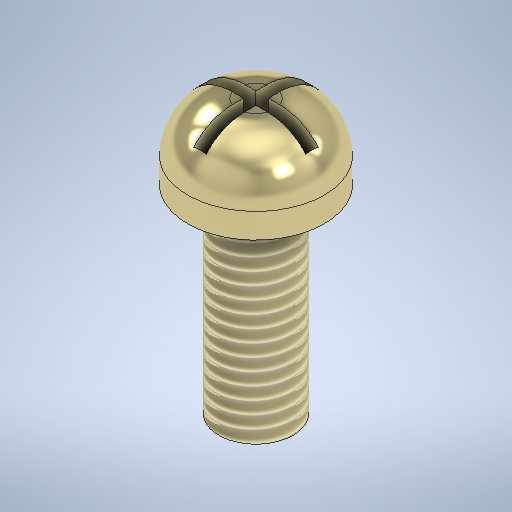
# Autodesk Inventor part: M3 Schraube
Saved by Autodesk Inventor 2025.1 (Build 291241000, 241)
## iProperties
Created: 2024-12-19
Part Number: M3 Schraube
Material: Generisch
Document SubType Name: Modeling
Designer: Julian
Density: 1 g/cm^3
Appearance: Vorgabe
Author: Julian
Autodesk Inventor part; units mm, degrees
ref_plane "YZ Plane" through (0, 0, 0) normal (1, 0, 0) x (0, 1, 0)
ref_plane "XZ Plane" through (0, 0, 0) normal (0, 1, 0) x (-1, 0, 0)
ref_plane "XY Plane" through (0, 0, 0) normal (0, 0, 1) x (1, 0, 0)
sketch "Skizze1" plane through (0, 0, 0) normal (0, 0, 1) x (1, 0, 0)
  circle A0 centre (0, 0) radius 2.75
  dimension "d0" = 5.5
  constraints: 1 centre point, 1 coincident
  measures "d0" diameter of A0
extrude "Extrusion1" add sketch "Skizze1" along normal blind 3
fillet "Rundung1" radius 2 1 edges at (-2.75, 0, 3)
sketch "Skizze2" plane through (0, 0, 3) normal (0, 0, 1) x (1, 0, 0)
  line L0 (0.25, -2.25) -> (-0.25, -2.25)
  line L1 (-0.25, 2.25) -> (0.25, 2.25)
  line L2 (0.25, -2.25) -> (-0.25, 2.25) construction
  line L3 (-0.25, -2.25) -> (0.25, 2.25) construction
  line L4 (-2.25, 0.25) -> (-2.25, -0.25)
  line L5 (2.25, -0.25) -> (2.25, 0.25)
  line L6 (2.25, 0.25) -> (-2.25, -0.25) construction
  line L7 (-2.25, 0.25) -> (2.25, -0.25) construction
  line L8 (-0.25, 0.25) -> (-2.25, 0.25)
  line L9 (-0.25, 0.25) -> (-0.25, 2.25)
  line L10 (-0.25, -2.25) -> (-0.25, -0.25)
  line L11 (-0.25, -0.0278) -> (-0.25, 0.0278)
  line L12 (2.25, 0.25) -> (0.25, 0.25)
  line L13 (0.0278, 0.25) -> (-0.0278, 0.25)
  line L14 (0.25, -0.25) -> (2.25, -0.25)
  line L15 (-2.25, -0.25) -> (-0.25, -0.25)
  line L16 (-0.0278, -0.25) -> (0.0278, -0.25)
  line L17 (0.25, -0.25) -> (0.25, -2.25)
  line L18 (0.25, 2.25) -> (0.25, 0.25)
  line L19 (0.25, 0.0278) -> (0.25, -0.0278)
  point P0 (0, 0)
  dimension "d4" = 0.5
  dimension "d5" = 4.5
  dimension "d6" = 4.5
  dimension "d7" = 0.5
  constraints: 40 end point, 20 parallel, 8 point on line, 6 perpendicular, 4 horizontal, 4 midpoint
  measures "d4" distance of L1.start L1.end
  measures "d5" distance of L0.end L1.start
  measures "d6" distance of L5.start L4.end
  measures "d7" distance of L4.end L4.start
extrude "Extrusion2" cut sketch "Skizze2" against normal blind 1.5
sketch "Skizze3" plane through (0, 0, 0) normal (0, 0, -1) x (-1, 0, 0)
  circle A0 centre (0, 0) radius 1.5
  dimension "d10" = 3
  constraints: 1 centre point, 1 coincident
  measures "d10" diameter of A0
extrude "Extrusion3" add sketch "Skizze3" along normal blind 8
thread "Gewinde1" size "M3x0.5" class "6g" standard "ANSI Metric M Profile" full length
